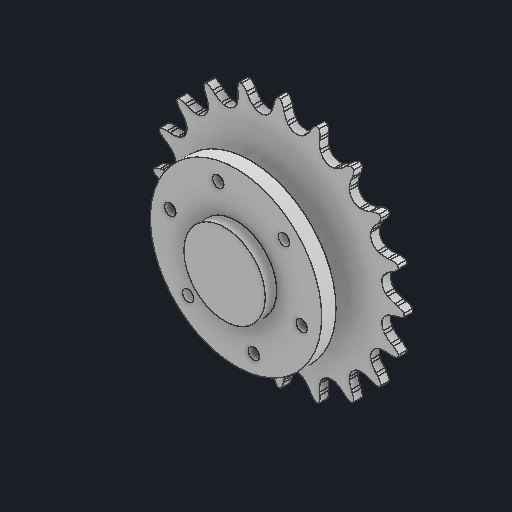
# Autodesk Inventor part: LegHubMY6812
Saved by Autodesk Inventor 2025.2 (Build 292293000, 293)
## iProperties
Created: 2025-10-06
Part Number: LegHubMY6812
Material: Generic
Document SubType Name: Modeling
Designer: valer
Density: 1 g/cm^3
Appearance: Default
Author: valer
Autodesk Inventor part; units mm, degrees
ref_plane "YZ Plane" through (0, 0, 0) normal (1, 0, 0) x (0, 1, 0)
ref_plane "XZ Plane" through (0, 0, 0) normal (0, 1, 0) x (-1, 0, 0)
ref_plane "XY Plane" through (0, 0, 0) normal (0, 0, 1) x (1, 0, 0)
sketch "Sketch1" plane through (0, 0, 0) normal (0, 0, 1) x (1, 0, 0)
  circle A0 centre (0, 0) radius 30
  dimension "d0" = 60
  constraints: 1 centre point, 1 coincident
  measures "d0" diameter of A0
extrude "Extrusion1" add sketch "Sketch1" along normal blind 5
sketch "Sketch2" plane through (0, 0, 5) normal (0, 0, 1) x (1, 0, 0)
  circle A0 centre (6.2371, -22.9812) radius 1.9939
  circle A1 centre (23.0208, -6.0891) radius 1.9939
  circle A2 centre (-23.0208, 6.0891) radius 1.9939
  circle A3 centre (-16.7837, -16.8921) radius 1.9939
  circle A4 centre (-6.2371, 22.9812) radius 1.9939
  circle A5 centre (16.7837, 16.8921) radius 1.9939
  circle A6 centre (0, 0) radius 14.2875 construction
  point P0 (0, 0)
extrude "Extrusion2" cut sketch "Sketch2" against normal through all
sketch "Sketch6" plane through (0, 0, 0) normal (0, 0, -1) x (-1, 0, 0)
  circle A0 centre (0, 0) radius 30 projected
  circle A1 centre (0, 0) radius 7.5
  dimension "d13" = 15
  constraints: 1 centre point, 1 coincident
  measures "d13" diameter of A1
extrude "Extrusion6" add sketch "Sketch6" along normal blind 10 contours A1
sketch "Sketch7" plane through (0, 0, 5) normal (0, 0, 1) x (1, 0, 0)
  circle A0 centre (0, 0) radius 14.25
  dimension "d16" = 28.5
  constraints: 1 centre point, 1 coincident
  measures "d16" diameter of A0
extrude "Extrusion7" add sketch "Sketch7" along normal blind 4
sketch "Sketch8" plane through (0, 0, -10) normal (0, 0, -1) x (-1, 0, 0)
  spline S0 degree 3 poles (35.8463, 25.3467) (35.6862, 24.8642) (35.4671, 24.395) (35.0284, 23.6883) (34.8404, 23.4299) (34.6359, 23.1879) knots 1.786806 1.786806 1.786806 1.786806 1.936294 1.936294 2.029294 2.029294 2.029294 2.029294
  arc A0 (35.8463, 25.3467) -> (35.1832, 26.2593) centre (0, 0) ccw
  spline S1 degree 3 poles (32.7561, 25.7752) (33.0494, 25.8949) (33.3533, 25.9939) (34.1609, 26.1927) (34.6749, 26.2562) (35.1832, 26.2593) knots 0.186373 0.186373 0.186373 0.186373 0.279373 0.279373 0.428862 0.428862 0.428862 0.428862
  line L0 (31.8448, 25.4034) -> (32.7561, 25.7752)
  spline S2 degree 3 poles (29.1929, 24.7126) (29.8864, 24.7977) (30.5859, 24.9563) (31.4571, 25.2519) (31.6523, 25.3248) (31.8448, 25.4034) knots -4.212131 -4.212131 -4.212131 -4.212131 -4.007748 -4.007748 -3.947883 -3.947883 -3.947883 -3.947883
  spline S3 degree 3 poles (28.2817, 24.7048) (28.3479, 24.6978) (28.4137, 24.6925) (28.711, 24.6759) (28.9518, 24.683) (29.1929, 24.7126) knots -1.623802 -1.623802 -1.623802 -1.623802 -1.603911 -1.603911 -1.533022 -1.533022 -1.533022 -1.533022
  spline S4 degree 3 poles (32.5242, 20.1275) (32.4215, 19.9073) (32.3404, 19.6806) (32.2643, 19.3926) (32.249, 19.3284) (32.2351, 19.2633) knots 0.221601 0.221601 0.221601 0.221601 0.292489 0.292489 0.312381 0.312381 0.312381 0.312381
  spline S5 degree 3 poles (34.0006, 22.4361) (33.8665, 22.2774) (33.7368, 22.1142) (33.1864, 21.377) (32.8194, 20.7607) (32.5242, 20.1275) knots 0.282089 0.282089 0.282089 0.282089 0.341955 0.341955 0.546337 0.546337 0.546337 0.546337
  line L1 (34.6359, 23.1879) -> (34.0006, 22.4361)
  spline S6 degree 3 poles (41.9245, 13.029) (41.6231, 12.6196) (41.2696, 12.2411) (40.6341, 11.7045) (40.3754, 11.5168) (40.1061, 11.3499) knots 1.786806 1.786806 1.786806 1.786806 1.936294 1.936294 2.029294 2.029294 2.029294 2.029294
  arc A1 (41.9245, 13.029) -> (41.5758, 14.1019) centre (0, 0) ccw
  spline S7 degree 3 poles (39.1178, 14.3915) (39.4338, 14.4147) (39.7534, 14.415) (40.5829, 14.3545) (41.0914, 14.256) (41.5758, 14.1019) knots 0.186373 0.186373 0.186373 0.186373 0.279373 0.279373 0.428862 0.428862 0.428862 0.428862
  line L2 (38.1363, 14.3194) -> (39.1178, 14.3915)
  spline S8 degree 3 poles (35.4007, 14.482) (36.0866, 14.3487) (36.8008, 14.2832) (37.7207, 14.2952) (37.929, 14.3042) (38.1363, 14.3194) knots -4.212131 -4.212131 -4.212131 -4.212131 -4.007748 -4.007748 -3.947883 -3.947883 -3.947883 -3.947883
  spline S9 degree 3 poles (34.5316, 14.7561) (34.5925, 14.729) (34.6534, 14.7037) (34.9311, 14.596) (35.1622, 14.5283) (35.4007, 14.482) knots -1.623802 -1.623802 -1.623802 -1.623802 -1.603911 -1.603911 -1.533022 -1.533022 -1.533022 -1.533022
  spline S10 degree 3 poles (37.1521, 9.0918) (36.9864, 8.9142) (36.8392, 8.7236) (36.6778, 8.4732) (36.6434, 8.4169) (36.6101, 8.3592) knots 0.221601 0.221601 0.221601 0.221601 0.292489 0.292489 0.312381 0.312381 0.312381 0.312381
  spline S11 degree 3 poles (39.2696, 10.8313) (39.093, 10.7217) (38.9192, 10.6066) (38.168, 10.0756) (37.6286, 9.6028) (37.1521, 9.0918) knots 0.282089 0.282089 0.282089 0.282089 0.341955 0.341955 0.546337 0.546337 0.546337 0.546337
  line L3 (40.1061, 11.3499) -> (39.2696, 10.8313)
  spline S12 degree 3 poles (43.8987, -0.5641) (43.4855, -0.8603) (43.0324, -1.1111) (42.2622, -1.425) (41.9582, -1.5235) (41.6505, -1.5991) knots 1.786806 1.786806 1.786806 1.786806 1.936294 1.936294 2.029294 2.029294 2.029294 2.029294
  arc A2 (43.8987, -0.5641) -> (43.8987, 0.5641) centre (0, 0) ccw
  spline S13 degree 3 poles (41.6505, 1.5991) (41.9582, 1.5235) (42.2622, 1.425) (43.0324, 1.1111) (43.4855, 0.8603) (43.8987, 0.5641) knots 0.186373 0.186373 0.186373 0.186373 0.279373 0.279373 0.428862 0.428862 0.428862 0.428862
  line L4 (40.6947, 1.8339) -> (41.6505, 1.5991)
  spline S14 degree 3 poles (38.1432, 2.8338) (38.7543, 2.495) (39.4134, 2.2121) (40.292, 1.9392) (40.4928, 1.8834) (40.6947, 1.8339) knots -4.212131 -4.212131 -4.212131 -4.212131 -4.007748 -4.007748 -3.947883 -3.947883 -3.947883 -3.947883
  spline S15 degree 3 poles (37.4014, 3.363) (37.4509, 3.3185) (37.501, 3.2755) (37.7319, 3.0873) (37.9308, 2.9515) (38.1432, 2.8338) knots -1.623802 -1.623802 -1.623802 -1.623802 -1.603911 -1.603911 -1.533022 -1.533022 -1.533022 -1.533022
  spline S16 degree 3 poles (38.1432, -2.8338) (37.9308, -2.9515) (37.7319, -3.0873) (37.501, -3.2755) (37.4509, -3.3185) (37.4014, -3.363) knots 0.221601 0.221601 0.221601 0.221601 0.292489 0.292489 0.312381 0.312381 0.312381 0.312381
  spline S17 degree 3 poles (40.6947, -1.8339) (40.4928, -1.8834) (40.292, -1.9392) (39.4134, -2.2121) (38.7543, -2.495) (38.1432, -2.8338) knots 0.282089 0.282089 0.282089 0.282089 0.341955 0.341955 0.546337 0.546337 0.546337 0.546337
  line L5 (41.6505, -1.5991) -> (40.6947, -1.8339)
  spline S18 degree 3 poles (41.5758, -14.1019) (41.0914, -14.256) (40.5829, -14.3545) (39.7534, -14.415) (39.4338, -14.4147) (39.1178, -14.3915) knots 1.786806 1.786806 1.786806 1.786806 1.936294 1.936294 2.029294 2.029294 2.029294 2.029294
  arc A3 (41.5758, -14.1019) -> (41.9245, -13.029) centre (0, 0) ccw
  spline S19 degree 3 poles (40.1061, -11.3499) (40.3754, -11.5168) (40.6341, -11.7045) (41.2696, -12.2411) (41.6231, -12.6196) (41.9245, -13.029) knots 0.186373 0.186373 0.186373 0.186373 0.279373 0.279373 0.428862 0.428862 0.428862 0.428862
  line L6 (39.2696, -10.8313) -> (40.1061, -11.3499)
  spline S20 degree 3 poles (37.1521, -9.0918) (37.6286, -9.6028) (38.168, -10.0756) (38.9192, -10.6066) (39.093, -10.7217) (39.2696, -10.8313) knots -4.212131 -4.212131 -4.212131 -4.212131 -4.007748 -4.007748 -3.947883 -3.947883 -3.947883 -3.947883
  spline S21 degree 3 poles (36.6101, -8.3592) (36.6434, -8.4169) (36.6778, -8.4732) (36.8392, -8.7236) (36.9864, -8.9142) (37.1521, -9.0918) knots 0.837373 0.837373 0.837373 0.837373 0.857264 0.857264 0.928153 0.928153 0.928153 0.928153
  spline S22 degree 3 poles (35.4007, -14.482) (35.1622, -14.5283) (34.9311, -14.596) (34.6534, -14.7037) (34.5925, -14.729) (34.5316, -14.7561) knots 0.221601 0.221601 0.221601 0.221601 0.292489 0.292489 0.312381 0.312381 0.312381 0.312381
  spline S23 degree 3 poles (38.1363, -14.3194) (37.929, -14.3042) (37.7207, -14.2952) (36.8008, -14.2832) (36.0866, -14.3487) (35.4007, -14.482) knots 0.282089 0.282089 0.282089 0.282089 0.341955 0.341955 0.546337 0.546337 0.546337 0.546337
  line L7 (39.1178, -14.3915) -> (38.1363, -14.3194)
  spline S24 degree 3 poles (35.1832, -26.2593) (34.6749, -26.2562) (34.1609, -26.1927) (33.3533, -25.9939) (33.0494, -25.8949) (32.7561, -25.7752) knots 1.786806 1.786806 1.786806 1.786806 1.936294 1.936294 2.029294 2.029294 2.029294 2.029294
  arc A4 (35.1832, -26.2593) -> (35.8463, -25.3467) centre (0, 0) ccw
  spline S25 degree 3 poles (34.6359, -23.1879) (34.8404, -23.4299) (35.0284, -23.6883) (35.4671, -24.395) (35.6862, -24.8642) (35.8463, -25.3467) knots 0.186373 0.186373 0.186373 0.186373 0.279373 0.279373 0.428862 0.428862 0.428862 0.428862
  line L8 (34.0006, -22.4361) -> (34.6359, -23.1879)
  spline S26 degree 3 poles (32.5242, -20.1275) (32.8194, -20.7607) (33.1864, -21.377) (33.7368, -22.1142) (33.8665, -22.2774) (34.0006, -22.4361) knots -4.212131 -4.212131 -4.212131 -4.212131 -4.007748 -4.007748 -3.947883 -3.947883 -3.947883 -3.947883
  spline S27 degree 3 poles (32.2351, -19.2633) (32.249, -19.3284) (32.2643, -19.3926) (32.3404, -19.6806) (32.4215, -19.9073) (32.5242, -20.1275) knots -1.623802 -1.623802 -1.623802 -1.623802 -1.603911 -1.603911 -1.533022 -1.533022 -1.533022 -1.533022
  spline S28 degree 3 poles (29.1929, -24.7126) (28.9518, -24.683) (28.711, -24.6759) (28.4137, -24.6925) (28.3479, -24.6978) (28.2817, -24.7048) knots 0.221601 0.221601 0.221601 0.221601 0.292489 0.292489 0.312381 0.312381 0.312381 0.312381
  spline S29 degree 3 poles (31.8448, -25.4034) (31.6523, -25.3248) (31.4571, -25.2519) (30.5859, -24.9563) (29.8864, -24.7977) (29.1929, -24.7126) knots 0.282089 0.282089 0.282089 0.282089 0.341955 0.341955 0.546337 0.546337 0.546337 0.546337
  line L9 (32.7561, -25.7752) -> (31.8448, -25.4034)
  spline S30 degree 3 poles (25.3467, -35.8463) (24.8642, -35.6862) (24.395, -35.4671) (23.6883, -35.0284) (23.4299, -34.8404) (23.1879, -34.6359) knots 1.786806 1.786806 1.786806 1.786806 1.936294 1.936294 2.029294 2.029294 2.029294 2.029294
  arc A5 (25.3467, -35.8463) -> (26.2593, -35.1832) centre (0, 0) ccw
  spline S31 degree 3 poles (25.7752, -32.7561) (25.8949, -33.0494) (25.9939, -33.3533) (26.1927, -34.1609) (26.2562, -34.6749) (26.2593, -35.1832) knots 0.186373 0.186373 0.186373 0.186373 0.279373 0.279373 0.428862 0.428862 0.428862 0.428862
  line L10 (25.4034, -31.8448) -> (25.7752, -32.7561)
  spline S32 degree 3 poles (24.7126, -29.1929) (24.7977, -29.8864) (24.9563, -30.5859) (25.2519, -31.4571) (25.3248, -31.6523) (25.4034, -31.8448) knots -4.212131 -4.212131 -4.212131 -4.212131 -4.007748 -4.007748 -3.947883 -3.947883 -3.947883 -3.947883
  spline S33 degree 3 poles (24.7048, -28.2817) (24.6978, -28.3479) (24.6925, -28.4137) (24.6759, -28.711) (24.683, -28.9518) (24.7126, -29.1929) knots -1.623802 -1.623802 -1.623802 -1.623802 -1.603911 -1.603911 -1.533022 -1.533022 -1.533022 -1.533022
  spline S34 degree 3 poles (20.1275, -32.5242) (19.9073, -32.4215) (19.6806, -32.3404) (19.3926, -32.2643) (19.3284, -32.249) (19.2633, -32.2351) knots 0.221601 0.221601 0.221601 0.221601 0.292489 0.292489 0.312381 0.312381 0.312381 0.312381
  spline S35 degree 3 poles (22.4361, -34.0006) (22.2774, -33.8665) (22.1142, -33.7368) (21.377, -33.1864) (20.7607, -32.8195) (20.1275, -32.5242) knots 0.282089 0.282089 0.282089 0.282089 0.341955 0.341955 0.546337 0.546337 0.546337 0.546337
  line L11 (23.1879, -34.6359) -> (22.4361, -34.0006)
  spline S36 degree 3 poles (13.029, -41.9245) (12.6196, -41.6231) (12.2411, -41.2696) (11.7045, -40.6341) (11.5168, -40.3754) (11.3499, -40.1061) knots 1.786806 1.786806 1.786806 1.786806 1.936294 1.936294 2.029294 2.029294 2.029294 2.029294
  arc A6 (13.029, -41.9245) -> (14.1019, -41.5758) centre (0, 0) ccw
  spline S37 degree 3 poles (14.3915, -39.1178) (14.4147, -39.4338) (14.415, -39.7534) (14.3545, -40.5829) (14.256, -41.0914) (14.1019, -41.5758) knots 0.186373 0.186373 0.186373 0.186373 0.279373 0.279373 0.428862 0.428862 0.428862 0.428862
  line L12 (14.3194, -38.1363) -> (14.3915, -39.1178)
  spline S38 degree 3 poles (14.482, -35.4007) (14.3487, -36.0866) (14.2832, -36.8008) (14.2952, -37.7207) (14.3042, -37.929) (14.3194, -38.1363) knots -4.212131 -4.212131 -4.212131 -4.212131 -4.007748 -4.007748 -3.947883 -3.947883 -3.947883 -3.947883
  spline S39 degree 3 poles (14.7561, -34.5316) (14.729, -34.5925) (14.7037, -34.6534) (14.596, -34.9311) (14.5283, -35.1622) (14.482, -35.4007) knots -1.623802 -1.623802 -1.623802 -1.623802 -1.603911 -1.603911 -1.533022 -1.533022 -1.533022 -1.533022
  spline S40 degree 3 poles (9.0918, -37.1521) (8.9142, -36.9864) (8.7236, -36.8392) (8.4732, -36.6778) (8.4169, -36.6434) (8.3592, -36.6101) knots 0.221601 0.221601 0.221601 0.221601 0.292489 0.292489 0.312381 0.312381 0.312381 0.312381
  spline S41 degree 3 poles (10.8313, -39.2696) (10.7217, -39.093) (10.6066, -38.9192) (10.0756, -38.168) (9.6028, -37.6286) (9.0918, -37.1521) knots 0.282089 0.282089 0.282089 0.282089 0.341955 0.341955 0.546337 0.546337 0.546337 0.546337
  line L13 (11.3499, -40.1061) -> (10.8313, -39.2696)
  spline S42 degree 3 poles (3.363, -37.4014) (3.3185, -37.4509) (3.2755, -37.501) (3.0873, -37.7319) (2.9515, -37.9308) (2.8338, -38.1432) knots -1.623802 -1.623802 -1.623802 -1.623802 -1.603911 -1.603911 -1.533022 -1.533022 -1.533022 -1.533022
  spline S43 degree 3 poles (-2.8338, -38.1432) (-2.9515, -37.9308) (-3.0873, -37.7319) (-3.2755, -37.501) (-3.3185, -37.4509) (-3.363, -37.4014) knots 0.221601 0.221601 0.221601 0.221601 0.292489 0.292489 0.312381 0.312381 0.312381 0.312381
  spline S44 degree 3 poles (-1.8339, -40.6947) (-1.8834, -40.4928) (-1.9392, -40.292) (-2.2121, -39.4134) (-2.495, -38.7543) (-2.8338, -38.1432) knots 0.282089 0.282089 0.282089 0.282089 0.341955 0.341955 0.546337 0.546337 0.546337 0.546337
  line L14 (-1.5991, -41.6505) -> (-1.8339, -40.6947)
  spline S45 degree 3 poles (-0.5641, -43.8987) (-0.8603, -43.4855) (-1.1111, -43.0324) (-1.425, -42.2622) (-1.5235, -41.9582) (-1.5991, -41.6505) knots 1.786806 1.786806 1.786806 1.786806 1.936294 1.936294 2.029294 2.029294 2.029294 2.029294
  arc A7 (-0.5641, -43.8987) -> (0.5641, -43.8987) centre (0, 0) ccw
  spline S46 degree 3 poles (1.5991, -41.6505) (1.5235, -41.9582) (1.425, -42.2622) (1.1111, -43.0324) (0.8603, -43.4855) (0.5641, -43.8987) knots 0.186373 0.186373 0.186373 0.186373 0.279373 0.279373 0.428862 0.428862 0.428862 0.428862
  line L15 (1.8339, -40.6947) -> (1.5991, -41.6505)
  spline S47 degree 3 poles (2.8338, -38.1432) (2.495, -38.7543) (2.2121, -39.4134) (1.9392, -40.292) (1.8834, -40.4928) (1.8339, -40.6947) knots -4.212131 -4.212131 -4.212131 -4.212131 -4.007748 -4.007748 -3.947883 -3.947883 -3.947883 -3.947883
  spline S48 degree 3 poles (-14.1019, -41.5758) (-14.256, -41.0914) (-14.3545, -40.5829) (-14.415, -39.7534) (-14.4147, -39.4338) (-14.3915, -39.1178) knots 1.786806 1.786806 1.786806 1.786806 1.936294 1.936294 2.029294 2.029294 2.029294 2.029294
  arc A8 (-14.1019, -41.5758) -> (-13.029, -41.9245) centre (0, 0) ccw
  spline S49 degree 3 poles (-11.3499, -40.1061) (-11.5168, -40.3754) (-11.7045, -40.6341) (-12.2411, -41.2696) (-12.6196, -41.6231) (-13.029, -41.9245) knots 0.186373 0.186373 0.186373 0.186373 0.279373 0.279373 0.428862 0.428862 0.428862 0.428862
  line L16 (-10.8313, -39.2696) -> (-11.3499, -40.1061)
  spline S50 degree 3 poles (-9.0918, -37.1521) (-9.6028, -37.6286) (-10.0756, -38.168) (-10.6066, -38.9192) (-10.7217, -39.093) (-10.8313, -39.2696) knots -4.212131 -4.212131 -4.212131 -4.212131 -4.007748 -4.007748 -3.947883 -3.947883 -3.947883 -3.947883
  spline S51 degree 3 poles (-8.3592, -36.6101) (-8.4169, -36.6434) (-8.4732, -36.6778) (-8.7236, -36.8392) (-8.9142, -36.9864) (-9.0918, -37.1521) knots 0.837373 0.837373 0.837373 0.837373 0.857264 0.857264 0.928153 0.928153 0.928153 0.928153
  spline S52 degree 3 poles (-14.482, -35.4007) (-14.5283, -35.1622) (-14.596, -34.9311) (-14.7037, -34.6534) (-14.729, -34.5925) (-14.7561, -34.5316) knots 0.221601 0.221601 0.221601 0.221601 0.292489 0.292489 0.312381 0.312381 0.312381 0.312381
  spline S53 degree 3 poles (-14.3194, -38.1363) (-14.3042, -37.929) (-14.2952, -37.7207) (-14.2833, -36.8008) (-14.3487, -36.0866) (-14.482, -35.4007) knots 0.282089 0.282089 0.282089 0.282089 0.341955 0.341955 0.546337 0.546337 0.546337 0.546337
  line L17 (-14.3915, -39.1178) -> (-14.3194, -38.1363)
  spline S54 degree 3 poles (-26.2593, -35.1832) (-26.2562, -34.6749) (-26.1927, -34.1609) (-25.9939, -33.3533) (-25.895, -33.0494) (-25.7752, -32.7561) knots 1.786806 1.786806 1.786806 1.786806 1.936294 1.936294 2.029294 2.029294 2.029294 2.029294
  arc A9 (-26.2593, -35.1832) -> (-25.3467, -35.8463) centre (0, 0) ccw
  spline S55 degree 3 poles (-23.1879, -34.6359) (-23.4299, -34.8404) (-23.6883, -35.0284) (-24.395, -35.4671) (-24.8642, -35.6862) (-25.3467, -35.8463) knots 0.186373 0.186373 0.186373 0.186373 0.279373 0.279373 0.428862 0.428862 0.428862 0.428862
  line L18 (-22.4361, -34.0006) -> (-23.1879, -34.6359)
  spline S56 degree 3 poles (-20.1275, -32.5242) (-20.7607, -32.8194) (-21.377, -33.1864) (-22.1142, -33.7368) (-22.2774, -33.8665) (-22.4361, -34.0006) knots -4.212131 -4.212131 -4.212131 -4.212131 -4.007748 -4.007748 -3.947883 -3.947883 -3.947883 -3.947883
  spline S57 degree 3 poles (-19.2633, -32.2351) (-19.3284, -32.249) (-19.3926, -32.2643) (-19.6806, -32.3404) (-19.9073, -32.4215) (-20.1275, -32.5242) knots -1.623802 -1.623802 -1.623802 -1.623802 -1.603911 -1.603911 -1.533022 -1.533022 -1.533022 -1.533022
  spline S58 degree 3 poles (-24.7126, -29.1929) (-24.683, -28.9518) (-24.6759, -28.711) (-24.6925, -28.4137) (-24.6978, -28.3479) (-24.7048, -28.2817) knots 0.221601 0.221601 0.221601 0.221601 0.292489 0.292489 0.312381 0.312381 0.312381 0.312381
  spline S59 degree 3 poles (-25.4034, -31.8448) (-25.3248, -31.6523) (-25.2519, -31.4571) (-24.9563, -30.5859) (-24.7977, -29.8864) (-24.7126, -29.1929) knots 0.282089 0.282089 0.282089 0.282089 0.341955 0.341955 0.546337 0.546337 0.546337 0.546337
  line L19 (-25.7752, -32.7561) -> (-25.4034, -31.8448)
  spline S60 degree 3 poles (-35.8463, -25.3467) (-35.6862, -24.8642) (-35.4671, -24.395) (-35.0284, -23.6883) (-34.8404, -23.4299) (-34.6359, -23.1879) knots 1.786806 1.786806 1.786806 1.786806 1.936294 1.936294 2.029294 2.029294 2.029294 2.029294
  arc A10 (-35.8463, -25.3467) -> (-35.1832, -26.2593) centre (0, 0) ccw
  spline S61 degree 3 poles (-32.7561, -25.7752) (-33.0494, -25.8949) (-33.3533, -25.9939) (-34.1609, -26.1927) (-34.6749, -26.2562) (-35.1832, -26.2593) knots 0.186373 0.186373 0.186373 0.186373 0.279373 0.279373 0.428862 0.428862 0.428862 0.428862
  line L20 (-31.8448, -25.4034) -> (-32.7561, -25.7752)
  spline S62 degree 3 poles (-29.1929, -24.7126) (-29.8864, -24.7977) (-30.5859, -24.9563) (-31.4571, -25.2519) (-31.6523, -25.3248) (-31.8448, -25.4034) knots -4.212131 -4.212131 -4.212131 -4.212131 -4.007748 -4.007748 -3.947883 -3.947883 -3.947883 -3.947883
  spline S63 degree 3 poles (-28.2817, -24.7048) (-28.3479, -24.6978) (-28.4137, -24.6925) (-28.711, -24.6759) (-28.9518, -24.683) (-29.1929, -24.7126) knots -1.623802 -1.623802 -1.623802 -1.623802 -1.603911 -1.603911 -1.533022 -1.533022 -1.533022 -1.533022
  spline S64 degree 3 poles (-32.5242, -20.1275) (-32.4215, -19.9073) (-32.3404, -19.6806) (-32.2643, -19.3926) (-32.249, -19.3284) (-32.2351, -19.2633) knots 0.221601 0.221601 0.221601 0.221601 0.292489 0.292489 0.312381 0.312381 0.312381 0.312381
  spline S65 degree 3 poles (-34.0006, -22.4361) (-33.8665, -22.2774) (-33.7368, -22.1142) (-33.1864, -21.377) (-32.8195, -20.7607) (-32.5242, -20.1275) knots 0.282089 0.282089 0.282089 0.282089 0.341955 0.341955 0.546337 0.546337 0.546337 0.546337
  line L21 (-34.6359, -23.1879) -> (-34.0006, -22.4361)
  spline S66 degree 3 poles (-41.9245, -13.029) (-41.6231, -12.6196) (-41.2696, -12.2411) (-40.6341, -11.7045) (-40.3754, -11.5168) (-40.1061, -11.3499) knots 1.786806 1.786806 1.786806 1.786806 1.936294 1.936294 2.029294 2.029294 2.029294 2.029294
  arc A11 (-41.9245, -13.029) -> (-41.5758, -14.1019) centre (0, 0) ccw
  spline S67 degree 3 poles (-39.1178, -14.3915) (-39.4338, -14.4147) (-39.7534, -14.415) (-40.5829, -14.3545) (-41.0914, -14.256) (-41.5758, -14.1019) knots 0.186373 0.186373 0.186373 0.186373 0.279373 0.279373 0.428862 0.428862 0.428862 0.428862
  line L22 (-38.1363, -14.3194) -> (-39.1178, -14.3915)
  spline S68 degree 3 poles (-35.4007, -14.482) (-36.0866, -14.3487) (-36.8008, -14.2832) (-37.7207, -14.2952) (-37.929, -14.3042) (-38.1363, -14.3194) knots -4.212131 -4.212131 -4.212131 -4.212131 -4.007748 -4.007748 -3.947883 -3.947883 -3.947883 -3.947883
  spline S69 degree 3 poles (-34.5316, -14.7561) (-34.5925, -14.729) (-34.6534, -14.7037) (-34.9311, -14.596) (-35.1622, -14.5283) (-35.4007, -14.482) knots -1.623802 -1.623802 -1.623802 -1.623802 -1.603911 -1.603911 -1.533022 -1.533022 -1.533022 -1.533022
  spline S70 degree 3 poles (-37.1521, -9.0918) (-36.9864, -8.9142) (-36.8392, -8.7236) (-36.6778, -8.4732) (-36.6434, -8.4169) (-36.6101, -8.3592) knots 0.221601 0.221601 0.221601 0.221601 0.292489 0.292489 0.312381 0.312381 0.312381 0.312381
  spline S71 degree 3 poles (-39.2696, -10.8313) (-39.093, -10.7217) (-38.9192, -10.6066) (-38.168, -10.0756) (-37.6286, -9.6028) (-37.1521, -9.0918) knots 0.282089 0.282089 0.282089 0.282089 0.341955 0.341955 0.546337 0.546337 0.546337 0.546337
  line L23 (-40.1061, -11.3499) -> (-39.2696, -10.8313)
  spline S72 degree 3 poles (-38.1432, 2.8338) (-37.9308, 2.9515) (-37.7319, 3.0873) (-37.501, 3.2755) (-37.4509, 3.3185) (-37.4014, 3.363) knots 0.221601 0.221601 0.221601 0.221601 0.292489 0.292489 0.312381 0.312381 0.312381 0.312381
  spline S73 degree 3 poles (-40.6947, 1.8339) (-40.4928, 1.8834) (-40.292, 1.9392) (-39.4134, 2.2121) (-38.7543, 2.495) (-38.1432, 2.8338) knots 0.282089 0.282089 0.282089 0.282089 0.341955 0.341955 0.546337 0.546337 0.546337 0.546337
  line L24 (-41.6505, 1.5991) -> (-40.6947, 1.8339)
  spline S74 degree 3 poles (-43.8987, 0.5641) (-43.4855, 0.8603) (-43.0324, 1.1111) (-42.2622, 1.425) (-41.9582, 1.5235) (-41.6505, 1.5991) knots 1.786806 1.786806 1.786806 1.786806 1.936294 1.936294 2.029294 2.029294 2.029294 2.029294
  arc A12 (-43.8987, 0.5641) -> (-43.8987, -0.5641) centre (0, 0) ccw
  spline S75 degree 3 poles (-41.6505, -1.5991) (-41.9582, -1.5235) (-42.2622, -1.425) (-43.0324, -1.1111) (-43.4855, -0.8603) (-43.8987, -0.5641) knots 0.186373 0.186373 0.186373 0.186373 0.279373 0.279373 0.428862 0.428862 0.428862 0.428862
  line L25 (-40.6947, -1.8339) -> (-41.6505, -1.5991)
  spline S76 degree 3 poles (-38.1432, -2.8338) (-38.7543, -2.495) (-39.4134, -2.2121) (-40.292, -1.9392) (-40.4928, -1.8834) (-40.6947, -1.8339) knots -4.212131 -4.212131 -4.212131 -4.212131 -4.007748 -4.007748 -3.947883 -3.947883 -3.947883 -3.947883
  spline S77 degree 3 poles (-37.4014, -3.363) (-37.4509, -3.3185) (-37.501, -3.2755) (-37.7319, -3.0873) (-37.9308, -2.9515) (-38.1432, -2.8338) knots -1.623802 -1.623802 -1.623802 -1.623802 -1.603911 -1.603911 -1.533022 -1.533022 -1.533022 -1.533022
  spline S78 degree 3 poles (-41.5758, 14.1019) (-41.0914, 14.256) (-40.5829, 14.3545) (-39.7534, 14.415) (-39.4338, 14.4147) (-39.1178, 14.3915) knots 1.786806 1.786806 1.786806 1.786806 1.936294 1.936294 2.029294 2.029294 2.029294 2.029294
  arc A13 (-41.5758, 14.1019) -> (-41.9245, 13.029) centre (0, 0) ccw
  spline S79 degree 3 poles (-40.1061, 11.3499) (-40.3754, 11.5168) (-40.6341, 11.7045) (-41.2696, 12.2411) (-41.6231, 12.6196) (-41.9245, 13.029) knots 0.186373 0.186373 0.186373 0.186373 0.279373 0.279373 0.428862 0.428862 0.428862 0.428862
  line L26 (-39.2696, 10.8313) -> (-40.1061, 11.3499)
  spline S80 degree 3 poles (-37.1521, 9.0918) (-37.6286, 9.6028) (-38.168, 10.0756) (-38.9192, 10.6066) (-39.093, 10.7217) (-39.2696, 10.8313) knots -4.212131 -4.212131 -4.212131 -4.212131 -4.007748 -4.007748 -3.947883 -3.947883 -3.947883 -3.947883
  spline S81 degree 3 poles (-36.6101, 8.3592) (-36.6434, 8.4169) (-36.6778, 8.4732) (-36.8392, 8.7236) (-36.9864, 8.9142) (-37.1521, 9.0918) knots 0.837373 0.837373 0.837373 0.837373 0.857264 0.857264 0.928153 0.928153 0.928153 0.928153
  spline S82 degree 3 poles (-35.4007, 14.482) (-35.1622, 14.5283) (-34.9311, 14.596) (-34.6534, 14.7037) (-34.5925, 14.729) (-34.5316, 14.7561) knots 0.221601 0.221601 0.221601 0.221601 0.292489 0.292489 0.312381 0.312381 0.312381 0.312381
  spline S83 degree 3 poles (-38.1363, 14.3194) (-37.929, 14.3042) (-37.7207, 14.2952) (-36.8008, 14.2832) (-36.0866, 14.3487) (-35.4007, 14.482) knots 0.282089 0.282089 0.282089 0.282089 0.341955 0.341955 0.546337 0.546337 0.546337 0.546337
  line L27 (-39.1178, 14.3915) -> (-38.1363, 14.3194)
  spline S84 degree 3 poles (-35.1832, 26.2593) (-34.6749, 26.2562) (-34.1609, 26.1927) (-33.3533, 25.9939) (-33.0494, 25.8949) (-32.7561, 25.7752) knots 1.786806 1.786806 1.786806 1.786806 1.936294 1.936294 2.029294 2.029294 2.029294 2.029294
  arc A14 (-35.1832, 26.2593) -> (-35.8463, 25.3467) centre (0, 0) ccw
  spline S85 degree 3 poles (-34.6359, 23.1879) (-34.8404, 23.4299) (-35.0284, 23.6883) (-35.4671, 24.395) (-35.6862, 24.8642) (-35.8463, 25.3467) knots 0.186373 0.186373 0.186373 0.186373 0.279373 0.279373 0.428862 0.428862 0.428862 0.428862
  line L28 (-34.0006, 22.4361) -> (-34.6359, 23.1879)
  spline S86 degree 3 poles (-32.5242, 20.1275) (-32.8194, 20.7607) (-33.1864, 21.377) (-33.7368, 22.1142) (-33.8665, 22.2774) (-34.0006, 22.4361) knots -4.212131 -4.212131 -4.212131 -4.212131 -4.007748 -4.007748 -3.947883 -3.947883 -3.947883 -3.947883
  spline S87 degree 3 poles (-32.2351, 19.2633) (-32.249, 19.3284) (-32.2643, 19.3926) (-32.3404, 19.6806) (-32.4215, 19.9073) (-32.5242, 20.1275) knots -1.623802 -1.623802 -1.623802 -1.623802 -1.603911 -1.603911 -1.533022 -1.533022 -1.533022 -1.533022
  spline S88 degree 3 poles (-29.1929, 24.7126) (-28.9518, 24.683) (-28.711, 24.6759) (-28.4137, 24.6925) (-28.3479, 24.6978) (-28.2817, 24.7048) knots 0.221601 0.221601 0.221601 0.221601 0.292489 0.292489 0.312381 0.312381 0.312381 0.312381
  spline S89 degree 3 poles (-31.8448, 25.4034) (-31.6523, 25.3248) (-31.4571, 25.2519) (-30.5859, 24.9563) (-29.8864, 24.7977) (-29.1929, 24.7126) knots 0.282089 0.282089 0.282089 0.282089 0.341955 0.341955 0.546337 0.546337 0.546337 0.546337
  line L29 (-32.7561, 25.7752) -> (-31.8448, 25.4034)
  spline S90 degree 3 poles (-25.3467, 35.8463) (-24.8642, 35.6862) (-24.395, 35.4671) (-23.6883, 35.0284) (-23.4299, 34.8404) (-23.1879, 34.6359) knots 1.786806 1.786806 1.786806 1.786806 1.936294 1.936294 2.029294 2.029294 2.029294 2.029294
  arc A15 (-25.3467, 35.8463) -> (-26.2593, 35.1832) centre (0, 0) ccw
  spline S91 degree 3 poles (-25.7752, 32.7561) (-25.8949, 33.0494) (-25.9939, 33.3533) (-26.1927, 34.1609) (-26.2562, 34.6749) (-26.2593, 35.1832) knots 0.186373 0.186373 0.186373 0.186373 0.279373 0.279373 0.428862 0.428862 0.428862 0.428862
  line L30 (-25.4034, 31.8448) -> (-25.7752, 32.7561)
  spline S92 degree 3 poles (-24.7126, 29.1929) (-24.7977, 29.8864) (-24.9563, 30.5859) (-25.2519, 31.4571) (-25.3248, 31.6523) (-25.4034, 31.8448) knots -4.212131 -4.212131 -4.212131 -4.212131 -4.007748 -4.007748 -3.947883 -3.947883 -3.947883 -3.947883
  spline S93 degree 3 poles (-24.7048, 28.2817) (-24.6978, 28.3479) (-24.6925, 28.4137) (-24.6759, 28.711) (-24.683, 28.9518) (-24.7126, 29.1929) knots -1.623802 -1.623802 -1.623802 -1.623802 -1.603911 -1.603911 -1.533022 -1.533022 -1.533022 -1.533022
  spline S94 degree 3 poles (-20.1275, 32.5242) (-19.9073, 32.4215) (-19.6806, 32.3404) (-19.3926, 32.2643) (-19.3284, 32.249) (-19.2633, 32.2351) knots 0.221601 0.221601 0.221601 0.221601 0.292489 0.292489 0.312381 0.312381 0.312381 0.312381
  spline S95 degree 3 poles (-22.4361, 34.0006) (-22.2774, 33.8665) (-22.1142, 33.7368) (-21.377, 33.1864) (-20.7607, 32.8194) (-20.1275, 32.5242) knots 0.282089 0.282089 0.282089 0.282089 0.341955 0.341955 0.546337 0.546337 0.546337 0.546337
  line L31 (-23.1879, 34.6359) -> (-22.4361, 34.0006)
  spline S96 degree 3 poles (-13.029, 41.9245) (-12.6196, 41.6231) (-12.2411, 41.2696) (-11.7045, 40.6341) (-11.5168, 40.3754) (-11.3499, 40.1061) knots 1.786806 1.786806 1.786806 1.786806 1.936294 1.936294 2.029294 2.029294 2.029294 2.029294
  arc A16 (-13.029, 41.9245) -> (-14.1019, 41.5758) centre (0, 0) ccw
  spline S97 degree 3 poles (-14.3915, 39.1178) (-14.4147, 39.4338) (-14.415, 39.7534) (-14.3545, 40.5829) (-14.256, 41.0914) (-14.1019, 41.5758) knots 0.186373 0.186373 0.186373 0.186373 0.279373 0.279373 0.428862 0.428862 0.428862 0.428862
  line L32 (-14.3194, 38.1363) -> (-14.3915, 39.1178)
  spline S98 degree 3 poles (-14.482, 35.4007) (-14.3487, 36.0866) (-14.2832, 36.8008) (-14.2952, 37.7207) (-14.3042, 37.929) (-14.3194, 38.1363) knots -4.212131 -4.212131 -4.212131 -4.212131 -4.007748 -4.007748 -3.947883 -3.947883 -3.947883 -3.947883
  spline S99 degree 3 poles (-14.7561, 34.5316) (-14.729, 34.5925) (-14.7037, 34.6534) (-14.596, 34.9311) (-14.5283, 35.1622) (-14.482, 35.4007) knots -1.623802 -1.623802 -1.623802 -1.623802 -1.603911 -1.603911 -1.533022 -1.533022 -1.533022 -1.533022
  spline S100 degree 3 poles (-9.0918, 37.1521) (-8.9142, 36.9864) (-8.7236, 36.8392) (-8.4732, 36.6778) (-8.4169, 36.6434) (-8.3592, 36.6101) knots 0.221601 0.221601 0.221601 0.221601 0.292489 0.292489 0.312381 0.312381 0.312381 0.312381
  spline S101 degree 3 poles (-10.8313, 39.2696) (-10.7217, 39.093) (-10.6066, 38.9192) (-10.0756, 38.168) (-9.6028, 37.6286) (-9.0918, 37.1521) knots 0.282089 0.282089 0.282089 0.282089 0.341955 0.341955 0.546337 0.546337 0.546337 0.546337
  line L33 (-11.3499, 40.1061) -> (-10.8313, 39.2696)
  spline S102 degree 3 poles (0.5641, 43.8987) (0.8603, 43.4855) (1.1111, 43.0324) (1.425, 42.2622) (1.5235, 41.9582) (1.5991, 41.6505) knots 1.786806 1.786806 1.786806 1.786806 1.936294 1.936294 2.029294 2.029294 2.029294 2.029294
  arc A17 (0.5641, 43.8987) -> (-0.5641, 43.8987) centre (0, 0) ccw
  spline S103 degree 3 poles (-1.5991, 41.6505) (-1.5235, 41.9582) (-1.425, 42.2622) (-1.1111, 43.0324) (-0.8603, 43.4855) (-0.5641, 43.8987) knots 0.186373 0.186373 0.186373 0.186373 0.279373 0.279373 0.428862 0.428862 0.428862 0.428862
  line L34 (-1.8339, 40.6947) -> (-1.5991, 41.6505)
  spline S104 degree 3 poles (-2.8338, 38.1432) (-2.495, 38.7543) (-2.2121, 39.4134) (-1.9392, 40.292) (-1.8834, 40.4928) (-1.8339, 40.6947) knots -4.212131 -4.212131 -4.212131 -4.212131 -4.007748 -4.007748 -3.947883 -3.947883 -3.947883 -3.947883
  spline S105 degree 3 poles (-3.363, 37.4014) (-3.3185, 37.4509) (-3.2755, 37.501) (-3.0873, 37.7319) (-2.9515, 37.9308) (-2.8338, 38.1432) knots -1.623802 -1.623802 -1.623802 -1.623802 -1.603911 -1.603911 -1.533022 -1.533022 -1.533022 -1.533022
  spline S106 degree 3 poles (2.8338, 38.1432) (2.9515, 37.9308) (3.0873, 37.7319) (3.2755, 37.501) (3.3185, 37.4509) (3.363, 37.4014) knots 0.221601 0.221601 0.221601 0.221601 0.292489 0.292489 0.312381 0.312381 0.312381 0.312381
  spline S107 degree 3 poles (1.8339, 40.6947) (1.8834, 40.4928) (1.9392, 40.292) (2.2121, 39.4134) (2.495, 38.7543) (2.8338, 38.1432) knots 0.282089 0.282089 0.282089 0.282089 0.341955 0.341955 0.546337 0.546337 0.546337 0.546337
  line L35 (1.5991, 41.6505) -> (1.8339, 40.6947)
  spline S108 degree 3 poles (14.1019, 41.5758) (14.256, 41.0914) (14.3545, 40.5829) (14.415, 39.7534) (14.4147, 39.4338) (14.3915, 39.1178) knots 1.786806 1.786806 1.786806 1.786806 1.936294 1.936294 2.029294 2.029294 2.029294 2.029294
  arc A18 (14.1019, 41.5758) -> (13.029, 41.9245) centre (0, 0) ccw
  spline S109 degree 3 poles (11.3499, 40.1061) (11.5168, 40.3754) (11.7045, 40.6341) (12.2411, 41.2696) (12.6196, 41.6231) (13.029, 41.9245) knots 0.186373 0.186373 0.186373 0.186373 0.279373 0.279373 0.428862 0.428862 0.428862 0.428862
  line L36 (10.8313, 39.2696) -> (11.3499, 40.1061)
  spline S110 degree 3 poles (9.0918, 37.1521) (9.6028, 37.6286) (10.0756, 38.168) (10.6066, 38.9192) (10.7217, 39.093) (10.8313, 39.2696) knots -4.212131 -4.212131 -4.212131 -4.212131 -4.007748 -4.007748 -3.947883 -3.947883 -3.947883 -3.947883
  spline S111 degree 3 poles (8.3592, 36.6101) (8.4169, 36.6434) (8.4732, 36.6778) (8.7236, 36.8392) (8.9142, 36.9864) (9.0918, 37.1521) knots 0.837373 0.837373 0.837373 0.837373 0.857264 0.857264 0.928153 0.928153 0.928153 0.928153
  spline S112 degree 3 poles (14.482, 35.4007) (14.5283, 35.1622) (14.596, 34.9311) (14.7037, 34.6534) (14.729, 34.5925) (14.7561, 34.5316) knots 0.221601 0.221601 0.221601 0.221601 0.292489 0.292489 0.312381 0.312381 0.312381 0.312381
  spline S113 degree 3 poles (14.3194, 38.1363) (14.3042, 37.929) (14.2952, 37.7207) (14.2832, 36.8008) (14.3487, 36.0866) (14.482, 35.4007) knots 0.282089 0.282089 0.282089 0.282089 0.341955 0.341955 0.546337 0.546337 0.546337 0.546337
  line L37 (14.3915, 39.1178) -> (14.3194, 38.1363)
  spline S114 degree 3 poles (26.2593, 35.1832) (26.2562, 34.6749) (26.1927, 34.1609) (25.9939, 33.3533) (25.8949, 33.0494) (25.7752, 32.7561) knots 1.786806 1.786806 1.786806 1.786806 1.936294 1.936294 2.029294 2.029294 2.029294 2.029294
  arc A19 (26.2593, 35.1832) -> (25.3467, 35.8463) centre (0, 0) ccw
  spline S115 degree 3 poles (23.1879, 34.6359) (23.4299, 34.8404) (23.6883, 35.0284) (24.395, 35.4671) (24.8642, 35.6862) (25.3467, 35.8463) knots 0.186373 0.186373 0.186373 0.186373 0.279373 0.279373 0.428862 0.428862 0.428862 0.428862
  line L38 (22.4361, 34.0006) -> (23.1879, 34.6359)
  spline S116 degree 3 poles (20.1275, 32.5242) (20.7607, 32.8195) (21.377, 33.1864) (22.1142, 33.7368) (22.2774, 33.8665) (22.4361, 34.0006) knots -4.212131 -4.212131 -4.212131 -4.212131 -4.007748 -4.007748 -3.947883 -3.947883 -3.947883 -3.947883
  spline S117 degree 3 poles (19.2633, 32.2351) (19.3284, 32.249) (19.3926, 32.2643) (19.6806, 32.3404) (19.9073, 32.4215) (20.1275, 32.5242) knots -1.623802 -1.623802 -1.623802 -1.623802 -1.603911 -1.603911 -1.533022 -1.533022 -1.533022 -1.533022
  spline S118 degree 3 poles (24.7126, 29.1929) (24.683, 28.9518) (24.6759, 28.711) (24.6925, 28.4137) (24.6978, 28.3479) (24.7048, 28.2817) knots 0.221601 0.221601 0.221601 0.221601 0.292489 0.292489 0.312381 0.312381 0.312381 0.312381
  spline S119 degree 3 poles (25.4034, 31.8448) (25.3248, 31.6523) (25.2519, 31.4571) (24.9563, 30.5859) (24.7977, 29.8864) (24.7126, 29.1929) knots 0.282089 0.282089 0.282089 0.282089 0.341955 0.341955 0.546337 0.546337 0.546337 0.546337
  line L39 (25.7752, 32.7561) -> (25.4034, 31.8448)
  arc A20 (8.3592, -36.6101) -> (3.363, -37.4014) centre (6.35, -40.0923) ccw
  arc A21 (19.2633, -32.2351) -> (14.7561, -34.5316) centre (18.4284, -36.1678) ccw
  arc A22 (28.2817, -24.7048) -> (24.7048, -28.2817) centre (28.7029, -28.7029) ccw
  arc A23 (34.5316, -14.7561) -> (32.2351, -19.2633) centre (36.1678, -18.4284) ccw
  arc A24 (37.4014, -3.363) -> (36.6101, -8.3592) centre (40.0923, -6.35) ccw
  arc A25 (36.6101, 8.3592) -> (37.4014, 3.363) centre (40.0923, 6.35) ccw
  arc A26 (32.2351, 19.2633) -> (34.5316, 14.7561) centre (36.1678, 18.4284) ccw
  arc A27 (24.7048, 28.2817) -> (28.2817, 24.7048) centre (28.7029, 28.7029) ccw
  arc A28 (14.7561, 34.5316) -> (19.2633, 32.2351) centre (18.4284, 36.1678) ccw
  arc A29 (3.363, 37.4014) -> (8.3592, 36.6101) centre (6.35, 40.0923) ccw
  arc A30 (-8.3592, 36.6101) -> (-3.363, 37.4014) centre (-6.35, 40.0923) ccw
  arc A31 (-19.2633, 32.2351) -> (-14.7561, 34.5316) centre (-18.4284, 36.1678) ccw
  arc A32 (-28.2817, 24.7048) -> (-24.7048, 28.2817) centre (-28.7029, 28.7029) ccw
  arc A33 (-34.5316, 14.7561) -> (-32.2351, 19.2633) centre (-36.1678, 18.4284) ccw
  arc A34 (-37.4014, 3.363) -> (-36.6101, 8.3592) centre (-40.0923, 6.35) ccw
  arc A35 (-36.6101, -8.3592) -> (-37.4014, -3.363) centre (-40.0923, -6.35) ccw
  arc A36 (-32.2351, -19.2633) -> (-34.5316, -14.7561) centre (-36.1678, -18.4284) ccw
  arc A37 (-24.7048, -28.2817) -> (-28.2817, -24.7048) centre (-28.7029, -28.7029) ccw
  arc A38 (-14.7561, -34.5316) -> (-19.2633, -32.2351) centre (-18.4284, -36.1678) ccw
  arc A39 (-3.363, -37.4014) -> (-8.3592, -36.6101) centre (-6.35, -40.0923) ccw
  circle A40 centre (0, 0) radius 43.9023 construction
  point P0 (28.2817, 24.7048)
  point P1 (24.7048, 28.2817)
  point P2 (14.7561, 34.5316)
  point P3 (3.363, 37.4014)
  point P4 (-8.3592, 36.6101)
  point P5 (-19.2633, 32.2351)
  point P6 (-37.4014, 3.363)
  point P7 (-37.4014, -3.363)
  point P8 (-32.2351, -19.2633)
  point P9 (-24.7048, -28.2817)
  point P10 (-19.2633, -32.2351)
  point P11 (-14.7561, -34.5316)
  point P12 (-8.3592, -36.6101)
  point P13 (3.363, -37.4014)
  point P14 (8.3592, -36.6101)
  point P15 (14.7561, -34.5316)
  point P16 (32.2351, -19.2633)
  point P17 (36.6101, -8.3592)
  point P18 (37.4014, -3.363)
  point P19 (36.6101, 8.3592)
  constraints: 80 end point, 80 point on circle, 61 centre point, 1 coincident, 360 other
extrude "Extrusion8" add sketch "Sketch8" along normal blind 3
sketch "Sketch9" plane through (0, 0, 0) normal (1, 0, 0) x (0, 1, 0)
  spline S0 degree 3 poles (-1.1241, -2.5746) (-0.8164, -2.4984) (-0.5124, -2.4234) (0.2578, -2.2333) (0.7109, -2.1216) (1.1241, -2.0193) knots 0.186373 0.186373 0.186373 0.186373 0.279373 0.279373 0.428862 0.428862 0.428862 0.428862
  line L0 (1.1241, -2.0193) -> (1.1241, 2.0193)
  spline S1 degree 3 poles (1.1241, 2.0193) (0.7109, 2.1216) (0.2578, 2.2333) (-0.5124, 2.4234) (-0.8164, 2.4984) (-1.1241, 2.5746) knots -0.428862 -0.428862 -0.428862 -0.428862 -0.279373 -0.279373 -0.186373 -0.186373 -0.186373 -0.186373
  spline S2 degree 3 poles (-1.1241, -2.5746) (-0.8164, -2.4984) (-0.5124, -2.4234) (0.2578, -2.2333) (0.7109, -2.1216) (1.1241, -2.0193) knots 0.186373 0.186373 0.186373 0.186373 0.279373 0.279373 0.428862 0.428862 0.428862 0.428862
  line L1 (1.1241, -2.0193) -> (1.1241, 2.0193)
  spline S3 degree 3 poles (1.1241, 2.0193) (0.7109, 2.1216) (0.2578, 2.2333) (-0.5124, 2.4234) (-0.8164, 2.4984) (-1.1241, 2.5746) knots -0.428862 -0.428862 -0.428862 -0.428862 -0.279373 -0.279373 -0.186373 -0.186373 -0.186373 -0.186373
  line L2 (-0.5641, -10) -> (-0.5641, -13) projected
  line L3 (-0.5641, -13) -> (-1.5991, -13) projected
  line L4 (-0.5641, -10) -> (-1.5991, -10) projected
  point P0 (0, 0)
  constraints: 4 end point, 12 other
body "Solid1"
